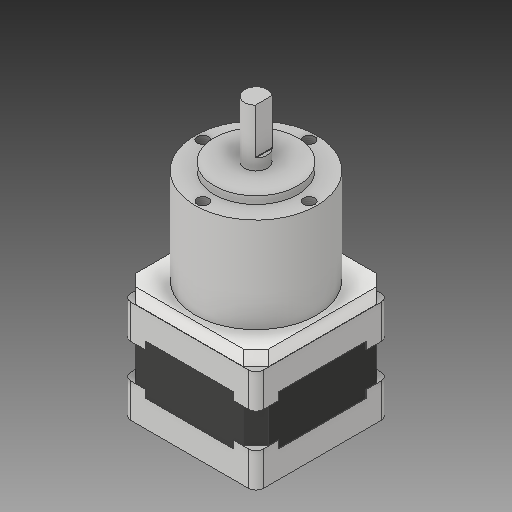
# Autodesk Inventor part: gearedstepper
Saved by Autodesk Inventor 2017 (Build 210142000, 142)
## iProperties
Created: 2016-04-04
Part Number: gearedstepper
Material: Generic
Document SubType Name: Modeling
Designer: brent
Density: 1 g/cm^3
Appearance: Default
Author: brent
Autodesk Inventor part; units mm, degrees
ref_plane "YZ Plane" through (0, 0, 0) normal (1, 0, 0) x (0, 1, 0)
ref_plane "XZ Plane" through (0, 0, 0) normal (0, 1, 0) x (-1, 0, 0)
ref_plane "XY Plane" through (0, 0, 0) normal (0, 0, 1) x (1, 0, 0)
sketch "Sketch1" plane through (0, 0, 0) normal (0, 1, 0) x (-1, 0, 0)
  circle A0 centre (0, 0) radius 3
  dimension "d0" = 6
  constraints: 1 centre point, 1 coincident
  measures "d0" diameter of A0
extrude "Extrusion1" add sketch "Sketch1" against normal blind 15
sketch "Sketch2" plane through (0, -15, 0) normal (0, -1, 0) x (1, 0, 0)
  circle A0 centre (0, 0) radius 11
  dimension "d3" = 22
  constraints: 1 centre point, 1 coincident
  measures "d3" diameter of A0
extrude "Extrusion2" add sketch "Sketch2" along normal blind 2
sketch "Sketch3" plane through (0, -17, 0) normal (0, -1, 0) x (1, 0, 0)
  circle A0 centre (0, 0) radius 16
  dimension "d6" = 32
  constraints: 1 centre point, 1 coincident
  measures "d6" diameter of A0
extrude "Extrusion3" add sketch "Sketch3" along normal blind 29
sketch "Sketch4" plane through (0, -46, 0) normal (0, -1, 0) x (1, 0, 0)
  line L0 (-17.4, 17.4) -> (17.4, 17.4)
  line L1 (17.4, 17.4) -> (17.4, -17.4)
  line L2 (17.4, -17.4) -> (-17.4, -17.4)
  line L3 (-17.4, -17.4) -> (-17.4, 17.4)
  line L4 (-17.4, 17.4) -> (17.4, -17.4) construction
  line L5 (17.4, 17.4) -> (-17.4, -17.4) construction
  point P0 (0, 0)
  dimension "d9" = 34.8
  dimension "d10" = 34.8
  constraints: 12 end point, 2 midpoint, 2 parallel, 1 horizontal, 1 perpendicular
  measures "d9" distance of L1.end L2.end
  measures "d10" distance of L0.end L1.end
extrude "Extrusion4" add sketch "Sketch4" against normal blind 4
chamfer "Chamfer1" distance 3.175 angle 45 4 edges at (17.4, -44, 17.4) (17.4, -44, -17.4) (-17.4, -44, 17.4) (-17.4, -44, -17.4)
sketch "Sketch5" plane through (0, -46, 0) normal (0, -1, 0) x (1, 0, 0)
  line L0 (17.5, -17.5) -> (-17.5, -17.5)
  line L1 (-17.5, -17.5) -> (-17.5, 17.5)
  line L2 (-17.5, 17.5) -> (17.5, 17.5)
  line L3 (17.5, 17.5) -> (17.5, -17.5)
  line L4 (17.5, -17.5) -> (-17.5, 17.5) construction
  line L5 (-17.5, -17.5) -> (17.5, 17.5) construction
  point P0 (0, 0)
  dimension "d16" = 35
  dimension "d17" = 35
  constraints: 12 end point, 2 midpoint, 2 parallel, 1 horizontal, 1 perpendicular
  measures "d16" distance of L1.end L2.end
  measures "d17" distance of L0.end L1.end
extrude "Extrusion5" add sketch "Sketch5" along normal blind 7
sketch "Sketch6" plane through (0, -53, 0) normal (0, -1, 0) x (1, 0, 0)
  line L0 (-17.5, 17.5) -> (-17.5, -17.5) projected
  line L1 (-17.5, -17.5) -> (17.5, -17.5) projected
  line L2 (17.5, -17.5) -> (17.5, 17.5) projected
  line L3 (17.5, 17.5) -> (-17.5, 17.5) projected
  line L4 (11.5, 17.5) -> (17.5, 17.5)
  line L5 (17.5, 17.5) -> (17.5, 11.5)
  line L6 (17.5, 11.5) -> (11.5, 11.5)
  line L7 (11.5, 11.5) -> (11.5, 17.5)
  circle A0 centre (0, 0) radius 16 projected
  circle A1 centre (0, 0) radius 16 projected
  line L8 (-17.5, 17.5) -> (-11.5, 17.5)
  line L9 (-17.5, 11.5) -> (-17.5, 17.5)
  line L10 (-11.5, 11.5) -> (-17.5, 11.5)
  line L11 (-11.5, 17.5) -> (-11.5, 11.5)
  line L12 (-17.5, -17.5) -> (-17.5, -11.5)
  line L13 (-11.5, -17.5) -> (-17.5, -17.5)
  line L14 (-11.5, -11.5) -> (-11.5, -17.5)
  line L15 (-17.5, -11.5) -> (-11.5, -11.5)
  line L16 (17.5, -17.5) -> (11.5, -17.5)
  line L17 (17.5, -11.5) -> (17.5, -17.5)
  line L18 (11.5, -11.5) -> (17.5, -11.5)
  line L19 (11.5, -17.5) -> (11.5, -11.5)
  dimension "d43" = 6
  dimension "d44" = 6
  dimension "d47" = 360
  constraints: 32 end point, 2 parallel, 2 point on line, 1 horizontal, 1 perpendicular, 33 other
  measures "d43" distance of L4.end L5.end
  measures "d44" distance of L4.start L4.end
extrude "Extrusion6" add sketch "Sketch6" along normal blind 2 contours L3 L11 L10 L0 | L15 L14 L1 L0 | L3 L2 L6 L7 | L19 L18 L2 L1
fillet "Fillet2" radius 2 4 edges at (17.5, -50.5, -17.5) (-17.5, -50.5, -17.5) (-17.5, -50.5, 17.5) (17.5, -50.5, 17.5)
sketch "Sketch7" plane through (0, -53, 0) normal (0, -1, 0) x (1, 0, 0)
  line L0 (-14.225, -17.4) -> (14.225, -17.4)
  line L1 (17.4, -14.225) -> (17.4, 14.225)
  line L2 (14.225, 17.4) -> (-14.225, 17.4)
  line L3 (-17.4, 14.225) -> (-17.4, -14.225)
  line L4 (-17.4, -17.4) -> (17.4, 17.4) construction
  line L5 (17.4, -17.4) -> (-17.4, 17.4) construction
  line L6 (-17.4, -14.225) -> (-14.225, -17.4)
  line L7 (14.225, -17.4) -> (17.4, -14.225)
  line L8 (17.4, 14.225) -> (14.225, 17.4)
  line L9 (-14.225, 17.4) -> (-17.4, 14.225)
  point P0 (0, 0)
  dimension "d31" = 34.8
  dimension "d32" = 34.8
  dimension "d33" = 3.175
  dimension "d34" = 3.175
  dimension "d35" = 3.175
  dimension "d36" = 3.175
  dimension "d37" = 3.175
  dimension "d38" = 3.175
  dimension "d39" = 3.175
  dimension "d40" = 3.175
  constraints: 20 end point, 8 point on line, 2 midpoint, 2 parallel, 1 horizontal, 1 perpendicular
  measures "d31" distance of L5.end L4.end
  measures "d32" distance of L4.end L5.start
  measures "d33" distance of L3.end L4.start
  measures "d34" distance of L0.start L4.start
  measures "d35" distance of L0.end L5.start
  measures "d36" distance of L1.start L5.start
  measures "d37" distance of L1.end L4.end
  measures "d38" distance of L2.start L4.end
  measures "d39" distance of L2.end L5.end
  measures "d40" distance of L3.start L5.end
extrude "Extrusion7" add sketch "Sketch7" along normal blind 6.5
mirror "Mirror1" about plane through (0, -59.5, 0) normal (0, -1, 0) of "Extrusion6", "Extrusion5", "Fillet2", "Extrusion7"
sketch "Sketch8" plane through (0, 0, 0) normal (0, 1, 0) x (1, 0, 0)
  circle A0 centre (0, 0) radius 3 projected
  line L0 (2, 2.2361) -> (2, -2.2361)
  dimension "d50" = 2
  constraints: 2 end point, 2 point on circle, 1 vertical
  measures "d50" distance from line of point (0, 0) L0
extrude "Extrusion8" cut sketch "Sketch8" against normal blind 12 contours A0 L0 picked at (2.1409, -0.5898)
fillet "Fillet3" radius 0.1 1 edges at (2, -12, 0)
sketch "Sketch9" plane through (0, -17, 0) normal (0, 1, 0) x (1, 0, 0)
  circle A0 centre (0, 0) radius 11 projected
  circle A1 centre (0, 0) radius 3 projected
  line L0 (0, 0) -> (0, -14) construction
  circle A2 centre (0, -14) radius 1.5
  dimension "d54" = 14
  dimension "d55" = 3
  constraints: 2 end point, 1 centre point, 1 coincident, 1 vertical
  measures "d54" distance of L0.start L0.end
  measures "d55" diameter of A2
extrude "Extrusion9" cut sketch "Sketch9" against normal blind 5 contours A2
thread "Thread1" size "M3x0.5" class "6H" standard "ANSI Metric M Profile" full length
pattern_circular "Circular Pattern1" count 4 over 360 about axis through (0, -17, 0) along (0, -1, 0) of "Extrusion9"
sketch "Sketch10" plane through (0, -17, 0) normal (0, 1, 0) x (1, 0, 0)
  point P0 (0, -14)
hole "Hole1" at (0, -17, 14) direction (0, -1, 0) diameter 2.459 depth 7.65 tip angle 120 thread size "M3x0.5" class "6H" standard "ANSI Metric M Profile"
equation "\"d34\" = d33"
equation "\"d35\" = d33"
equation "\"d36\" = d35"
equation "\"d37\" = d33"
equation "\"d38\" = d37"
equation "\"d39\" = d33"
equation "\"d40\" = d39"
body "Solid1"
